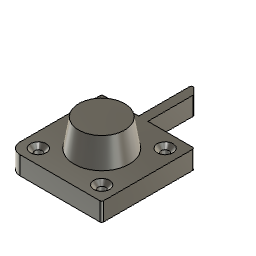
Base_Front_Right (Autodesk Fusion 360 design; units mm, degrees)
Autodesk Fusion 360 part; units mm, degrees
note: some values were not read from the file. Set by a fixed rule: which sketch regions a step uses.
sketch "Skizze1" plane through (0, 0, 0) normal (0, 0, 1) x (1, 0, 0)
  line L0 (0, 0) -> (50.5, 0)
  line L1 (50.5, 0) -> (50.5, 50.5)
  line L2 (50.5, 50.5) -> (0, 50.5)
  line L3 (0, 50.5) -> (0, 0)
  line L4 (0, 50.5) -> (20.1, 50.5)
  line L5 (20.1, 50.5) -> (20.1, 80.5)
  line L6 (20.1, 50.5) -> (25.1, 50.5)
  line L7 (25.1, 50.5) -> (25.1, 75.5)
  line L8 (25.1, 75.5) -> (20.1, 80.5)
  line L9 (50.5, 0) -> (50.5, 20.1)
  line L10 (50.5, 20.1) -> (50.5, 25.1)
  dimension "d1" = 50.5
  dimension "d2" = 50.5
  dimension "d3" = 20.1
  dimension "d4" = 30
  dimension "d5" = 5
  dimension "d6" = 25
  constraint horizontal L0
  constraint vertical L1
  constraint horizontal L2
  constraint vertical L3
  constraint coincident L0.start L3.end
  constraint perpendicular L3 L4
  constraint perpendicular L2 L5
  constraint perpendicular L5 L6
  constraint perpendicular L6 L7
  constraint perpendicular L0 L9
  measures "d1" distance of L0.start L0.end
  measures "d2" distance of L0.start L2.end
  measures "d3" distance of L2.end L4.end
  measures "d4" distance of L4.end L5.end
  measures "d5" distance of L4.end L6.end
  measures "d6" distance of L6.end L7.end
extrude "Extrusion1" add sketch "Skizze1" along normal blind 10
sketch "Skizze2" plane through (0, 0, 10) normal (0, 0, 1) x (-1, 0, 0)
  line L0 (-50.5, 0) -> (-50.5, -50.5)
  line L1 (-50.5, -50.5) -> (-25.1, -50.5)
  line L2 (-25.1, -50.5) -> (-25.1, -75.5)
  line L3 (-25.1, -75.5) -> (-20.1, -80.5)
  line L4 (-20.1, -80.5) -> (-20.1, -50.5)
  line L5 (-20.1, -50.5) -> (0, -50.5)
  line L6 (0, -50.5) -> (0, 0)
  line L7 (0, 0) -> (-50.5, 0)
  line L8 (-25.25, 0) -> (-25.25, -50.5)
  circle A0 centre (-25.25, -25.25) radius 15
  line L9 (0, 0) -> (0, -8)
  line L10 (0, -8) -> (-8, -8)
  line L11 (-50.5, 0) -> (-50.5, -8)
  line L12 (-50.5, -8) -> (-42.5, -8)
  line L13 (-50.5, -50.5) -> (-50.5, -42.5)
  line L14 (-50.5, -42.5) -> (-42.5, -42.5)
  line L15 (0, -50.5) -> (0, -42.5)
  line L16 (0, -42.5) -> (-8, -42.5)
  dimension "d13" = 30
  dimension "d14" = 8
  dimension "d15" = 8
  dimension "d16" = 8
  dimension "d17" = 8
  dimension "d18" = 8
  dimension "d19" = 8
  dimension "d20" = 8
  dimension "d21" = 8
  constraint midpoint L7 L8.start
  constraint coincident L1 L8.end
  constraint perpendicular L1 L8
  constraint midpoint L8 A0.centre
  constraint coincident L6.end L7.start
  constraint perpendicular L7 L9
  constraint perpendicular L9 L10
  constraint coincident L0.start L7.end
  constraint perpendicular L7 L11
  constraint perpendicular L11 L12
  constraint coincident L0.end L1.start
  constraint perpendicular L1 L13
  constraint perpendicular L13 L14
  constraint coincident L5.end L6.start
  constraint perpendicular L5 L15
  constraint perpendicular L6 L16
  measures "d13" diameter of A0
  measures "d14" distance of L6.end L9.end
  measures "d15" distance of L9.end L10.end
  measures "d16" distance of L0.start L11.end
  measures "d17" distance of L11.end L12.end
  measures "d18" distance of L0.end L13.end
  measures "d19" distance of L13.end L14.end
  measures "d20" distance of L5.end L15.end
  measures "d21" distance of L15.end L16.end
extrude "Extrusion2" add sketch "Skizze2" along normal blind 14.8 contours L8 A0 | L8 A0
chamfer "Fase1" distance 2.5 distance2 14.8 1 edges at (39.2349, 30.6742, 24.8) measured on face at (22.0767, 28.4139, 24.8)
hole "Bohrung1" at (8, 8, 10) direction (0, 0, -1) diameter 4.2 depth 13 tip angle 180 countersink diameter 8.6 countersink angle 90
hole "Bohrung2" at (42.5, 8, 10) at (42.5, 42.5, 10) at (8, 42.5, 10) direction (0, 0, -1) diameter 4.2 depth 13 tip angle 180 countersink diameter 8.6 countersink angle 90
fillet "Abrundung1" radius 6 1 edges at (0, 0, 5)
fillet "Abrundung2" radius 1 5 edges at (25.1, 75.5, 5) (20.1, 80.5, 5) (0, 50.5, 5) (50.5, 50.5, 5) (50.5, 0, 5)
